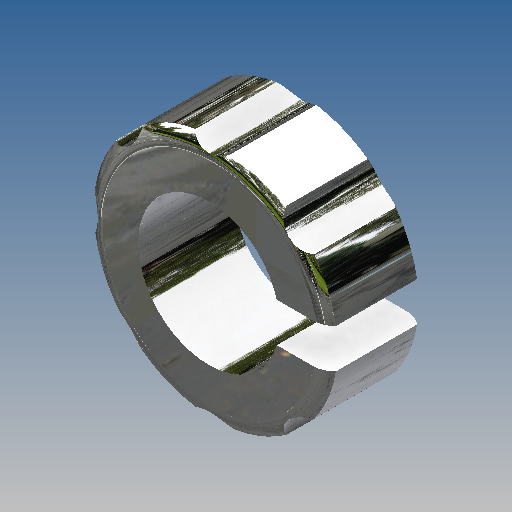
# Autodesk Inventor part: PWTR-0108
Saved by Autodesk Inventor 2021.1 (Build 251245000, 245)
## iProperties
Created: 2015-03-16
Part Number: PWTR-0108
Material: Aluminum 6061
Document SubType Name: Modeling
Designer: baris
Density: 2.7 g/cm^3
Appearance: Aluminum - Flat
Description: Level Adjustment Screw Collar
Author: baris
Revision Number: A
Autodesk Inventor part; units mm, degrees
ref_plane "YZ Plane" through (0, 0, 0) normal (1, 0, 0) x (0, 1, 0)
ref_plane "XZ Plane" through (0, 0, 0) normal (0, 1, 0) x (-1, 0, 0)
ref_plane "XY Plane" through (0, 0, 0) normal (0, 0, 1) x (1, 0, 0)
sketch "Sketch1" plane through (0, 0, 0) normal (0, 1, 0) x (-1, 0, 0)
  line L0 (-1.1714, -12.4618) -> (-1.1714, -27.4618) construction
  line L1 (8.1, -25.7) -> (8.1, -10.7) construction
  line L2 (-1.1714, -21.2152) -> (8.1, -21.2152) construction
  line L3 (3.4643, -21.2152) -> (3.4643, 9.1343) construction
  line L4 (-3.267, -19.9618) -> (-1.0357, -19.9618)
  line L5 (-1.0357, -19.9618) -> (-1.0357, -13.9618)
  line L6 (-1.0357, -13.9618) -> (-3.267, -13.9618)
  line L7 (-4.2857, -14.3912) -> (-4.2857, -19.5563)
  arc A0 (-4.2857, -19.5563) -> (-3.267, -19.9618) centre (-3.267, -18.4795) ccw
  arc A1 (-3.267, -13.9618) -> (-4.2857, -14.3912) centre (-3.267, -15.3848) ccw
  point P0 (0, 0)
  dimension "d0" = 7.75
  dimension "d1" = 4.5
  dimension "d2" = 6
  constraints: 16 end point, 4 point on circle, 2 centre point, 2 horizontal, 2 parallel, 2 point on line, 2 tangent, 2 vertical, 1 midpoint, 1 perpendicular, 2 other
  measures "d0" distance between parallel lines of L3 L7
  measures "d1" distance between parallel lines of L3 L5
  measures "d2" distance between parallel lines of L6 L4
revolve "Revolution1" add sketch "Sketch1" angle 360 about axis through (-3.4643, 0, -21.2152) along (0, 0, 1)
sketch "Sketch2" plane through (-3.4643, 0, -13.9618) normal (0, 0, 1) x (1, 0, 0)
  circle A0 centre (0.0167, -8.8653) radius 1.75
  circle A1 centre (6.2805, -6.2569) radius 1.75
  circle A2 centre (8.8653, 0.0167) radius 1.75
  circle A3 centre (6.2569, 6.2805) radius 1.75
  circle A4 centre (-0.0167, 8.8653) radius 1.75
  circle A5 centre (-6.2805, 6.2569) radius 1.75
  circle A6 centre (-8.8653, -0.0167) radius 1.75
  circle A7 centre (-6.2569, -6.2805) radius 1.75
  point P0 (3.4643, 0)
  point P1 (0, 0)
  dimension "d4" = 3.5
  dimension "d7" = 360
  constraints: 8 centre point, 17 other
  measures "d4" diameter of A0
extrude "Extrusion1" cut sketch "Sketch2" against normal blind 10 contours A0 | A1 | A3 | A4 | A5 | A6 | A7
sketch "Sketch3" plane through (-3.4643, 0, -13.9618) normal (0, 0, 1) x (1, 0, 0)
  line L0 (0, 0) -> (8.4123, 0) construction
  line L1 (8.4123, 0) -> (8.4123, -1.25)
  line L2 (8.4123, -1.25) -> (0, -1.25)
  line L3 (0, -1.25) -> (0, 0)
  line L4 (8.4123, 0) -> (8.4123, 1.25)
  line L5 (8.4123, 1.25) -> (0, 1.25)
  line L6 (0, 1.25) -> (0, 0)
  point P0 (3.4643, 0)
  dimension "d11" = 1.25
  constraints: 14 end point, 2 parallel, 2 symmetric about line, 1 horizontal, 1 perpendicular
  measures "d11" distance between parallel lines of L0 L2
extrude "Extrusion2" cut sketch "Sketch3" against normal blind 10
body "Solid1"
